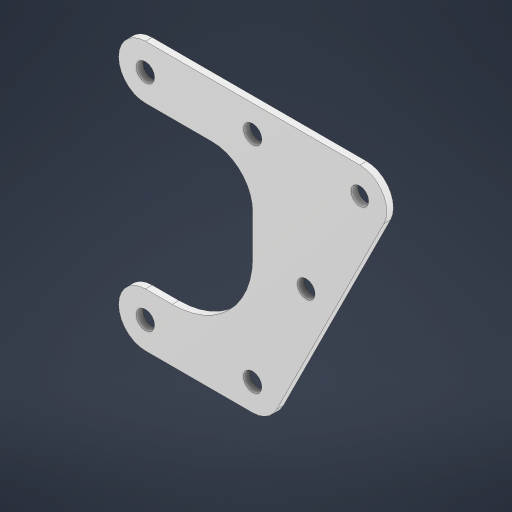
# Autodesk Inventor part: gusset
Saved by Autodesk Inventor 2024 (Build 280153000, 153)
## iProperties
Created: 2024-01-15
Part Number: gusset
Material: Acetal Resin, White
Document SubType Name: Modeling
Designer: avere
Density: 1.425 g/cm^3
Appearance: Smooth - White
d0: 0.500 in
d1: 0.500 in
d2: 0.172 in
d3: 0.750 in
d4: 0.375 in
d7: 0.172 in
d8: 0.165 in
d10: 0.165 in
Author: avere
Autodesk Inventor part; units mm, degrees
ref_plane "YZ Plane" through (0, 0, 0) normal (1, 0, 0) x (0, 1, 0)
ref_plane "XZ Plane" through (0, 0, 0) normal (0, 1, 0) x (-1, 0, 0)
ref_plane "XY Plane" through (0, 0, 0) normal (0, 0, 1) x (1, 0, 0)
sketch "main" plane through (0, 0, 0) normal (0, 0, 1) x (1, 0, 0)
  circle A0 centre (20.1733, 30.7236) radius 2.0955
  arc A1 (-24.2767, -13.7264) -> (-5.2267, 5.3236) centre (-24.2767, 5.3236) ccw
  line L0 (-5.2267, 14.8486) -> (-5.2267, 5.3236)
  line L1 (0.4529, -22.9162) -> (25.8529, 27.8838)
  arc A2 (-5.2267, 14.8486) -> (-14.7517, 24.3736) centre (-14.7517, 14.8486) ccw
  line L2 (-30.6267, 24.3736) -> (-14.7517, 24.3736)
  arc A3 (25.8529, 27.8838) -> (20.1733, 37.0736) centre (20.1733, 30.7236) ccw
  line L3 (20.1733, 37.0736) -> (-30.6267, 37.0736)
  circle A4 centre (-30.6267, 30.7236) radius 2.1844
  arc A5 (-30.6267, 37.0736) -> (-30.6267, 24.3736) centre (-30.6267, 30.7236) ccw
  line L4 (-30.6267, -13.7264) -> (-24.2767, -13.7264)
  circle A6 centre (-5.2267, -20.0764) radius 2.1844
  arc A7 (-5.2267, -26.4264) -> (0.4529, -22.9162) centre (-5.2267, -20.0764) ccw
  line L5 (-5.2267, -26.4264) -> (-30.6267, -26.4264)
  line L6 (-5.2267, -26.4264) -> (-30.6267, -26.4264)
  circle A8 centre (-30.6267, -20.0764) radius 2.1844
  arc A9 (-30.6267, -13.7264) -> (-30.6267, -26.4264) centre (-30.6267, -20.0764) ccw
  circle A10 centre (-5.2267, 30.7236) radius 2.1844
  circle A11 centre (7.4733, 5.3236) radius 2.0955
  point P0 (-10.623, 1.8831)
  point P1 (-5.2267, -13.7264)
  dimension "d0" = 12.7
  dimension "d1" = 12.7
  dimension "d2" = 4.3688
  dimension "d3" = 19.05
  dimension "d4" = 9.525
  dimension "d7" = 4.3688
  dimension "d8" = 4.191
  dimension "d10" = 4.191
  measures "d0" diameter of A3
  measures "d1" diameter of A7
  measures "d2" diameter of A8
  measures "d3" radius of A1
  measures "d4" radius of A2
  measures "d7" diameter of A10
  measures "d8" diameter of A11
  measures "d10" diameter of A0
sketch "Sketch1" plane through (0, 0, 0) normal (0, 0, 1) x (1, 0, 0)
  circle A0 centre (50.8, 0) radius 2.0955
  arc A1 (6.35, -44.45) -> (25.4, -25.4) centre (6.35, -25.4) ccw
  line L0 (25.4, -15.875) -> (25.4, -25.4)
  line L1 (31.0796, -53.6398) -> (56.4796, -2.8398)
  arc A2 (25.4, -15.875) -> (15.875, -6.35) centre (15.875, -15.875) ccw
  line L2 (0, -6.35) -> (15.875, -6.35)
  arc A3 (56.4796, -2.8398) -> (50.8, 6.35) centre (50.8, 0) ccw
  line L3 (50.8, 6.35) -> (0, 6.35)
  circle A4 centre (0, 0) radius 2.1844
  arc A5 (0, 6.35) -> (0, -6.35) centre (0, 0) ccw
  line L4 (0, -44.45) -> (6.35, -44.45)
  circle A6 centre (25.4, -50.8) radius 2.1844
  arc A7 (25.4, -57.15) -> (31.0796, -53.6398) centre (25.4, -50.8) ccw
  line L5 (25.4, -57.15) -> (0, -57.15)
  line L6 (25.4, -57.15) -> (0, -57.15)
  circle A8 centre (0, -50.8) radius 2.1844
  arc A9 (0, -44.45) -> (0, -57.15) centre (0, -50.8) ccw
  circle A10 centre (25.4, 0) radius 2.1844
  circle A11 centre (38.1, -25.4) radius 2.0955
  constraints: 1 other
extrude "Extrusion1" add sketch "Sketch1" along normal blind 1.5875
body "Solid1"
